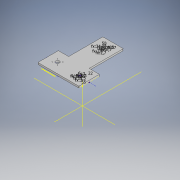
# Autodesk Inventor part: BT000_trajan20_21
Saved by Autodesk Inventor 2022.2 (Build 262287000, 287)
## iProperties
Company: HTBLA Kaindorf
RuleStatus: InUse
Created: 2022-05-24
Part Number: BT000_trajan20_21
Project: Zeichenmaschine_Inventor
Material: Generisch
Description: Masterskizze
Document SubType Name: Modeling
Designer: trajan20
Density: 1 g/cm^3
Appearance: Vorgabe
Mass: 519.269 g
Surface Area: 1176.66 cm^2
Volume: 519.269 cm^3
AfterDocNew0: iProperties-Editor_aufrufen
Zet_Kluppen_Höhe: 7,000 mm
Zet_KluppenDicke: 1,000 mm
Zet_Höhe: 5,000 mm
Zet_Kluppen_Breite: 10,000 mm
St_kurz_Breite: 10,000 mm
Zet_Breite: 210,000 mm
Gel_Mot_St_Breite: 10,000 mm
Gel_Mot_St_2: 35,000 mm
St_kurz_Höhe: 7,500 mm
Gel_Mot_St_Höhe: 5,000 mm
St_kurz_Länge: 140,000 mm
St_lang_Länge: 180,000 mm
Bas_Ver_Breite: 60,000 mm
Bas_Ver_Länge: 160,000 mm
Gel_Mot_St_1: 35,000 mm
SM_Pos_Abstand: 150,000 mm
GM_Halt_Höhe: 50,000 mm
Bas_Haupt_Höhe: 80,000 mm
Bas_Haupt_Breite: 80,000 mm
Bas_Haupt_Länge: 220,000 mm
Druck_teil_Höhe: 7,500 mm
Druck_teil_Durchmesser: 50,000 mm
Alu_Prof: 20,000 mm
Bas_Haupt_Plat_Höhe: 4,000 mm
SM_Scheibe_Durchmesser: 22,000 mm
SM_Schrauben_Pos_Abstand: 31,000 mm
GM_Platte_Höhe: 4,000 mm
Rundung_Platte: 2,000 mm
GM_Schrauben_Pos_Abstand_lang: 34,370 mm
GM_Stift_Durchmesser: 6,000 mm
GM_Schrauben_Pos_Abstand_kurz: 18,370 mm
GM_Schrauben_Durchgangsloch: 2,700 mm
GM_Schrauben_Pos_Stift_rlang: 9,050 mm
GM_Schrauben_Pos_Stift_rkurz: 9,185 mm
Author: jan
Keywords: 2021
Autodesk Inventor part; units mm, degrees
sketch "Basis" plane through (0, 0, 0) normal (0, 0, 1) x (1, 0, 0)
  line L0 (0, 150) -> (0, -150)
  line L1 (-79.5351, 0) -> (153.2558, 0) projected
  line L2 (0, -282) -> (0, 222) projected
  line L3 (30, -50) -> (30, -210)
  line L4 (0, -200) -> (20, -200)
  line L5 (0, -40) -> (120, -40)
  line L6 (0, 40) -> (120, 40)
  line L7 (110, -30) -> (110, 30)
  point P0 (0, 0)
  point P1 (110, 0)
  dimension "d32" = 300
  dimension "d38" = 80
  dimension "d39" = 10
  dimension "d40" = 10
  dimension "d41" = 10
  dimension "d43" = 240
  dimension "d44" = 240
  dimension "d45" = 60
  dimension "d46" = 10
  dimension "d47" = 10
  dimension "d48" = 160
  dimension "d49" = 10
  constraints: 12 end point, 6 point on line, 3 vertical, 2 midpoint, 2 perpendicular, 1 horizontal
  measures "d32" distance of L0.start L0.end
  measures "d38" distance between parallel lines of L5 L6
  measures "d39" distance from line of L5 L7.start
  measures "d40" distance from line of L5.end L7
  measures "d41" distance from line of L6 L7.end
  measures "d43" diameter of L5.end L0
  measures "d44" diameter of L6.end L0
  measures "d45" diameter of L3 L0
  measures "d46" distance from line of L3.end L4
  measures "d47" distance from line of L3 L4.end
  measures "d48" distance between parallel lines of L4 L5
  measures "d49" distance from line of L5 L3.start
ref_plane "Arbeitsebene7" through (120, 40, 0) normal (0, 1, 0) x (-1, 0, 0)
sketch "Skizze12" plane through (120, 40, 0) normal (0, 1, 0) x (-1, 0, 0)
  line L0 (10, -10) -> (10, -80)
  line L1 (20, -70) -> (120, -70)
  line L2 (120, -100.8) -> (120, 16.8) projected
  point P0 (120, 0)
  point P1 (10, 0)
  point P2 (10, 0)
  point P3 (10, 0)
  dimension "d50" = 70
  dimension "d51" = 10
  dimension "d80" = 10
  dimension "d81" = 10
  constraints: 4 end point, 2 point on line, 1 horizontal, 1 vertical
  measures "d50" distance of L0.start L0.end
  measures "d51" distance of point (10, 0) L0.start
  measures "d80" distance from line of L0 L1.start
  measures "d81" horizontal distance of L0.end L1.start
ref_plane "Arbeitsebene8" through (120, -40, 0) normal (0, 1, 0) x (-1, 0, 0)
sketch "Skizze13" plane through (120, -40, 0) normal (0, 1, 0) x (-1, 0, 0)
  line L0 (10, -10) -> (10, -80) projected
  line L1 (10, -10) -> (10, -80)
  line L2 (20, -70) -> (120, -70)
  line L3 (120, -100.8) -> (120, 16.8) projected
  point P0 (120, 0)
  dimension "d82" = 10
  dimension "d83" = 10
  constraints: 4 end point, 1 horizontal, 1 point on line, 1 vertical
  measures "d82" distance from line of L0 L2.start
  measures "d83" horizontal distance of L0.end L2.start
ref_plane "Arbeitsebene9" through (20, -200, 0) normal (0, -1, 0) x (1, 0, 0)
sketch "Skizze14" plane through (20, -200, 0) normal (0, -1, 0) x (1, 0, 0)
  line L0 (10, -10) -> (10, -50)
  point P0 (-20, 0)
  point P1 (10, 0)
  point P2 (10, 0)
  point P3 (10, 0)
  dimension "d52" = 40
  dimension "d53" = 10
  constraints: 2 end point, 1 point on line, 1 vertical
  measures "d52" distance of L0.start L0.end
  measures "d53" distance of point (10, 0) L0.start
ref_plane "Arbeitsebene10" through (20, -140, 0) normal (0, -1, 0) x (1, 0, 0)
sketch "Skizze15" plane through (20, -140, 0) normal (0, -1, 0) x (1, 0, 0)
  line L0 (10, -10) -> (10, -50) projected
  line L1 (10, -10) -> (10, -50)
  point P0 (-20, 0)
  constraints: 2 end point, 1 collinear
ref_plane "Arbeitsebene12" through (110, 40, -80) normal (1, 0, 0) x (0, 1, 0)
sketch "Skizze16" plane through (110, 40, -80) normal (1, 0, 0) x (0, 1, 0)
  line L0 (-90, 0) -> (10, 0)
  line L1 (10, 0) -> (10, -4)
  line L2 (10, -4) -> (-90, -4)
  line L3 (-90, -4) -> (-90, 0)
  line L4 (-70, 10) -> (-10, 10)
  line L5 (0, 70) -> (0, 0) projected
  line L6 (-80, 70) -> (-80, 0) projected
  point P0 (-40, 80)
  dimension "d66" = 4
  dimension "d67" = 10
  dimension "d68" = 10
  dimension "d77" = 10
  dimension "d78" = 10
  dimension "d79" = 10
  constraints: 10 end point, 2 horizontal, 2 parallel, 1 perpendicular, 1 point on line
  measures "d66" distance between parallel lines of L2 L0
  measures "d67" distance from line of L1 L5.end
  measures "d68" distance from line of L3 L6.end
  measures "d77" distance from line of L6 L4.start
  measures "d78" distance from line of L5 L4.end
  measures "d79" distance between parallel lines of L0 L4
ref_plane "Arbeitsebene17" through (110, -50, -84) normal (0, 0, 1) x (1, 0, 0)
sketch "Skizze18" plane through (110, -50, -84) normal (0, 0, 1) x (1, 0, 0)
  line L0 (-110, -232) -> (-110, 272) projected
  line L1 (-189.5351, 50) -> (43.2558, 50) projected
  line L2 (-19.5, 65.5) -> (-50.5, 65.5) construction
  line L3 (-50.5, 65.5) -> (-50.5, 34.5) construction
  line L4 (-19.5, 65.5) -> (-19.5, 34.5) construction
  line L5 (-19.5, 34.5) -> (-50.5, 34.5) construction
  point P0 (-110, 50)
  point P1 (-35, 50)
  dimension "d69" = 75
  dimension "d70" = 15.5
  dimension "d71" = 15.5
  dimension "d72" = 31
  dimension "d73" = 31
  constraints: 8 end point, 4 coincident, 2 perpendicular, 1 horizontal, 1 point on line, 1 vertical
  measures "d69" distance from line of L0 point (-35, 50)
  measures "d70" distance between parallel lines of L1 L2
  measures "d71" distance from line of L3 point (-35, 50)
  measures "d72" distance between parallel lines of L5 L2
  measures "d73" distance between parallel lines of L4 L3
ref_plane "Arbeitsebene18" through (30, -140, -50) normal (1, 0, 0) x (0, 1, 0)
sketch "Skizze19" plane through (30, -140, -50) normal (1, 0, 0) x (0, 1, 0)
  line L0 (10, -4) -> (-70, -4)
  line L1 (-70, -4) -> (-70, 0)
  line L2 (-70, 0) -> (10, 0)
  line L3 (10, 0) -> (10, -4)
  line L4 (-50, 10) -> (-10, 10)
  point P0 (140, 50)
  point P1 (-60, 0)
  point P2 (0, 0)
  dimension "d74" = 4
  dimension "d75" = 10
  dimension "d76" = 10
  dimension "d84" = 10
  dimension "d85" = 10
  dimension "d86" = 10
  constraints: 10 end point, 2 horizontal, 2 parallel, 1 perpendicular, 1 point on line
  measures "d74" distance between parallel lines of L0 L2
  measures "d75" distance from line of point (0, 0) L3
  measures "d76" distance from line of L1 point (-60, 0)
  measures "d84" horizontal distance of point (-60, 0) L4.start
  measures "d85" horizontal distance of point (-60, 0) L4.start
  measures "d86" horizontal distance of L4.end point (0, 0)
ref_plane "Arbeitsebene19" through (30, -210, -54) normal (0, 0, 1) x (1, 0, 0)
ref_plane "Arbeitsebene20" through (20, 2.5, 100) normal (0, 0, -1) x (-1, 0, 0)
sketch "Skizze 1" plane through (-280, -73.3, 100) normal (0, 0, 1) x (1, 0, 0)
  line L0 (-20, 13.3) -> (-20, 11.3) projected
  line L1 (180, 13.3) -> (-20, 13.3) projected
  line L2 (180, -106.7) -> (-20, -106.7) projected
  line L3 (-20, -104.7) -> (-20, -106.7) projected
  line L4 (180, 53.3) -> (180, -146.7) projected
  line L5 (180, 73.3) -> (180, -166.7) projected
  line L6 (300, 73.3) -> (300, -166.7) projected
  line L7 (180, 73.3) -> (182, 73.3) projected
  line L8 (298, 73.3) -> (300, 73.3) projected
  line L9 (300, -166.7) -> (298, -166.7) projected
  line L10 (182, -166.7) -> (180, -166.7) projected
  line L11 (-20, -106.7) -> (-20, 13.3) projected
  line L12 (180, 13.3) -> (-20, 13.3) projected
  line L13 (180, 13.3) -> (180, 73.3) projected
  line L14 (180, 73.3) -> (300, 73.3) projected
  line L15 (300, -166.7) -> (300, 73.3) projected
  line L16 (300, -166.7) -> (180, -166.7) projected
  line L17 (180, -166.7) -> (180, -106.7) projected
  line L18 (180, -106.7) -> (-20, -106.7) projected
extrude "Extrusion3" add sketch "Skizze 1" along normal blind 10
sketch "Skizze23" plane through (20, -242.5, 0) normal (1, 0, 0) x (0, 0, -1)
  line L0 (0, 245) -> (0, 0) projected
  line L1 (-100, 245) -> (0, 245) projected
  line L2 (0, 0) -> (-100, 0)
  line L3 (-100, 0) -> (-100, 245)
  line L4 (-100, 245) -> (0, 245)
  line L5 (0, 245) -> (0, 0)
  point P0 (0, 242.5)
  constraints: 8 end point, 2 parallel, 1 horizontal, 1 perpendicular
extrude "Extrusion4" cut sketch "Skizze23" against normal through all
sketch "Skizze20" plane through (30, -210, 100) normal (0, 0, 1) x (1, 0, 0)
  line L0 (0, 80) -> (0, 0) projected
  line L1 (-217.5819, 99.185) -> (-324.0785, 99.185) construction
  line L2 (-223.1225, 80.815) -> (-333.4519, 80.815) construction
  line L3 (-289.05, 125.855) -> (-289.05, 54.145) construction
  line L4 (-254.68, 148.5562) -> (-254.68, 51.145) construction
  line L5 (-44.2587, 170.5) -> (-93.3542, 170.5) construction
  line L6 (-85.5, 183.5563) -> (-85.5, 134.1968) construction
  line L7 (-97.1508, 139.5) -> (-51.7506, 139.5) construction
  line L8 (-54.5, 132.7748) -> (-54.5, 177.4853) construction
  line L9 (-327.4713, 90) -> (-3.4708, 90) construction
  line L10 (-70, 254.6178) -> (-70, -44.1957) construction
  line L11 (-130, 210) -> (-10, 210) construction
  line L12 (-330, 30) -> (-330, 150) construction
  circle A0 centre (-289.05, 99.185) radius 1.35
  circle A1 centre (-254.68, 99.185) radius 1.35
  circle A2 centre (-254.68, 80.815) radius 1.35
  circle A3 centre (-289.05, 80.815) radius 1.35
  circle A4 centre (-280, 90) radius 3
  circle A5 centre (-85.5, 170.5) radius 1.5
  circle A6 centre (-85.5, 139.5) radius 1.5
  circle A7 centre (-54.5, 139.5) radius 1.5
  circle A8 centre (-54.5, 170.5) radius 1.5
  circle A9 centre (-70, 155) radius 11
  point P0 (-30, 210)
  point P1 (-70, 210)
  point P2 (-330, 90)
  point P3 (-289.05, 90)
  dimension "d102" = 2.7
  dimension "d103" = 2.7
  dimension "d104" = 2.7
  dimension "d105" = 2.7
  dimension "d106" = 6
  dimension "d107" = 9.05
  dimension "d108" = 9.185
  dimension "d109" = 18.37
  dimension "d111" = 34.37
  dimension "d112" = 50
  dimension "d113" = 31
  dimension "d114" = 31
  dimension "d115" = 15.5
  dimension "d116" = 15.5
  dimension "d117" = 55
  dimension "d118" = 3
  dimension "d119" = 3
  dimension "d120" = 3
  dimension "d121" = 3
  dimension "d122" = 22
  constraints: 21 point on line, 20 end point, 10 centre point, 10 coincident, 5 horizontal, 3 midpoint, 3 vertical, 2 perpendicular
  measures "d102" diameter of A0
  measures "d103" diameter of A3
  measures "d104" diameter of A1
  measures "d105" diameter of A2
  measures "d106" diameter of A4
  measures "d107" horizontal distance of point (-289.05, 80.815) point (-280, 90)
  measures "d108" distance from line of point (-289.05, 80.815) L9
  measures "d109" distance between parallel lines of L1 L2
  measures "d111" distance between parallel lines of L3 L4
  measures "d112" distance from line of L12 point (-280, 90)
  measures "d113" distance between parallel lines of L7 L5
  measures "d114" distance between parallel lines of L6 L8
  measures "d115" distance from line of L7 point (-70, 155)
  measures "d116" distance from line of L8 point (-70, 155)
  measures "d117" distance from line of L11 point (-70, 155)
  measures "d118" diameter of A5
  measures "d119" diameter of A6
  measures "d120" diameter of A7
  measures "d121" diameter of A8
  measures "d122" diameter of A9
extrude "Extrusion5" cut sketch "Skizze20" along normal through all
ref_plane "Arbeitsebene21" through (-297.4713, -120, 100) normal (0, 1, 0) x (1, 0, 0)
mirror "Spiegeln1" about plane through (-297.4713, -120, 100) normal (0, 1, 0) of "Extrusion5"
fillet "Rundung1" radius 2 6 edges at (20, -240, 105) (20, 0, 105) (-100, 0, 105) (-300, -60, 105) (-300, -180, 105) (-100, -240, 105)
equation "\"d38\" = Bas_Haupt_Breite"
equation "\"d39\" = 0.5 * Alu_Prof"
equation "\"d40\" = d39"
equation "\"d41\" = d39"
equation "\"d43\" = Bas_Haupt_Länge + Alu_Prof"
equation "\"d44\" = d43"
equation "\"d45\" = Bas_Ver_Breite"
equation "\"d46\" = d39"
equation "\"d47\" = d39"
equation "\"d48\" = Bas_Ver_Länge"
equation "\"d49\" = d39"
equation "\"d50\" = Bas_Haupt_Höhe - 0.5 * Alu_Prof"
equation "\"d51\" = d39"
equation "\"d80\" = d51"
equation "\"d81\" = d51"
equation "\"d82\" = d81"
equation "\"d83\" = d81"
equation "\"d52\" = GM_Halt_Höhe - 0.5 * Alu_Prof"
equation "\"d53\" = d39"
equation "\"d66\" = Bas_Haupt_Plat_Höhe"
equation "\"d67\" = 0.5 * Alu_Prof"
equation "\"d68\" = d67"
equation "\"d77\" = d68"
equation "\"d78\" = d68"
equation "\"d79\" = d68"
equation "\"d69\" = 0.5 * SM_Pos_Abstand"
equation "\"d70\" = 0.5 * SM_Schrauben_Pos_Abstand"
equation "\"d71\" = d70"
equation "\"d72\" = SM_Schrauben_Pos_Abstand"
equation "\"d73\" = SM_Schrauben_Pos_Abstand"
equation "\"d74\" = GM_Platte_Höhe"
equation "\"d75\" = 0.5 * Alu_Prof"
equation "\"d76\" = d75"
equation "\"d84\" = d76"
equation "\"d85\" = d76"
equation "\"d86\" = d76"
equation "\"Zet_Kluppen_Höhe\" = 7"
equation "\"Zet_KluppenDicke\" = 1"
equation "\"Zet_Höhe\" = 5"
equation "\"Zet_Kluppen_Breite\" = 10"
equation "\"St_kurz_Breite\" = 10"
equation "\"Zet_Breite\" = 210"
equation "\"Gel_Mot_St_Breite\" = 10"
equation "\"Gel_Mot_St_2\" = 35"
equation "\"St_kurz_Höhe\" = 7.5"
equation "\"Gel_Mot_St_Höhe\" = 5"
equation "\"St_kurz_Länge\" = 140"
equation "\"St_lang_Länge\" = 180"
equation "\"Bas_Ver_Breite\" = 60"
equation "\"Bas_Ver_Länge\" = 160"
equation "\"Gel_Mot_St_1\" = 35"
equation "\"SM_Pos_Abstand\" = 150"
equation "\"GM_Halt_Höhe\" = 50"
equation "\"Bas_Haupt_Höhe\" = 80"
equation "\"Bas_Haupt_Breite\" = 80"
equation "\"Bas_Haupt_Länge\" = 220"
equation "\"Druck_teil_Höhe\" = 7.5"
equation "\"Druck_teil_Durchmesser\" = 50"
equation "\"Alu_Prof\" = 20"
equation "\"Bas_Haupt_Plat_Höhe\" = 4"
equation "\"SM_Scheibe_Durchmesser\" = 22"
equation "\"SM_Schrauben_Pos_Abstand\" = 31"
equation "\"GM_Platte_Höhe\" = 4"
equation "\"Rundung_Platte\" = 2"
equation "\"GM_Schrauben_Pos_Abstand_lang\" = 34.37"
equation "\"GM_Stift_Durchmesser\" = 6"
equation "\"GM_Schrauben_Pos_Abstand_kurz\" = 18.37"
equation "\"GM_Schrauben_Durchgangsloch\" = 2.7"
equation "\"GM_Schrauben_Pos_Stift_rlang\" = 9.05"
equation "\"GM_Schrauben_Pos_Stift_rkurz\" = 9.185"
